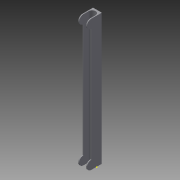
# Autodesk Inventor part: Filament Guide
Saved by Autodesk Inventor 2015 (Build 190159000, 159)
## iProperties
Created: 2014-08-31
Part Number: Filament Guide
Material: Generic
Document SubType Name: Modeling
Designer: Chris
Density: 1 g/cm^3
Appearance: Default
Author: Chris
Autodesk Inventor part; units mm, degrees
ref_plane "YZ Plane" through (0, 0, 0) normal (1, 0, 0) x (0, 1, 0)
ref_plane "XZ Plane" through (0, 0, 0) normal (0, 1, 0) x (-1, 0, 0)
ref_plane "XY Plane" through (0, 0, 0) normal (0, 0, 1) x (1, 0, 0)
sketch "Sketch3" plane through (0, 0, 0) normal (0, 0, 1) x (1, 0, 0)
  arc A0 (4, 0) -> (-4, 0) centre (0, 0) ccw
  line L0 (5, 0) -> (5, -6)
  line L1 (-5, -6) -> (-5, 0)
  line L2 (-4, 0) -> (-4, -6)
  line L3 (4, 0) -> (4, -6)
  line L4 (5, -6) -> (4, -6)
  line L5 (-4, -6) -> (-5, -6)
  line L6 (-5, 0) -> (-5, 6)
  line L7 (-5, 6) -> (5, 6)
  line L8 (5, 6) -> (5, 0)
  dimension "d9" = 8
  dimension "d11" = 6
  dimension "d29" = 10
  dimension "d30" = 6
  constraints: 18 end point, 4 perpendicular, 2 parallel, 2 point on circle, 2 tangent, 1 centre point, 1 coincident
  measures "d9" diameter of A0
  measures "d11" distance of L0.start L0.end
  measures "d29" distance of L6.end L7.end
  measures "d30" distance of L1.end L6.end
extrude "Extrusion3" add sketch "Sketch3" along normal blind 150
sketch "Sketch9" plane through (-5, -6, 0) normal (-1, 0, 0) x (0, 0, 1)
  line L0 (0, 0) -> (10, 0)
  line L1 (10, 0) -> (10, -5)
  line L2 (10, -5) -> (0, -5)
  line L3 (0, -5) -> (0, 0)
  point P0 (0, 6)
  dimension "d31" = 10
  dimension "d32" = 5
  constraints: 8 end point, 2 parallel, 1 horizontal, 1 perpendicular
  measures "d31" distance of L1.end L2.end
  measures "d32" distance of L0.end L1.end
extrude "Extrusion8" add sketch "Sketch9" against normal blind 1
sketch "Sketch10" plane through (-5, -6, 150) normal (-1, 0, 0) x (0, 0, 1)
  line L0 (0, 0) -> (-10, 0)
  line L1 (-10, 0) -> (-10, -5)
  line L2 (-10, -5) -> (0, -5)
  line L3 (0, -5) -> (0, 0)
  point P0 (-150, 6)
  dimension "d35" = 10
  dimension "d36" = 5
  constraints: 8 end point, 2 parallel, 1 horizontal, 1 perpendicular
  measures "d35" distance of L2.end L1.end
  measures "d36" distance of L1.end L0.end
extrude "Extrusion9" add sketch "Sketch10" against normal blind 1
sketch "Sketch11" plane through (5, -6, 0) normal (1, 0, 0) x (0, 0, -1)
  point P0 (0, 6)
sketch "Sketch12" plane through (5, -6, 0) normal (1, 0, 0) x (0, 0, -1)
  line L0 (0, 0) -> (-10, 0)
  line L1 (-10, 0) -> (-10, -5)
  line L2 (-10, -5) -> (0, -5)
  line L3 (0, -5) -> (0, 0)
  point P0 (0, 6)
  dimension "d39" = 10
  dimension "d40" = 5
  constraints: 8 end point, 2 parallel, 1 horizontal, 1 perpendicular
  measures "d39" distance of L2.end L1.end
  measures "d40" distance of L1.end L0.end
extrude "Extrusion10" add sketch "Sketch12" against normal blind 1
sketch "Sketch13" plane through (5, -6, 150) normal (1, 0, 0) x (0, 0, -1)
  line L0 (0, 0) -> (10, 0)
  line L1 (10, 0) -> (10, -5)
  line L2 (10, -5) -> (0, -5)
  line L3 (0, -5) -> (0, 0)
  point P0 (150, 6)
  dimension "d43" = 10
  dimension "d44" = 5
  constraints: 8 end point, 2 parallel, 1 horizontal, 1 perpendicular
  measures "d43" distance of L1.end L2.end
  measures "d44" distance of L0.end L1.end
extrude "Extrusion11" add sketch "Sketch13" against normal blind 1
fillet "Fillet4" radius 5 4 edges at (-4.5, -11, 150) (4.5, -11, 150) (-4.5, -11, 140) (4.5, -11, 140)
fillet "Fillet5" radius 5 4 edges at (4.5, -11, 0) (-4.5, -11, 0) (-4.5, -11, 10) (4.5, -11, 10)
body "Solid2"
